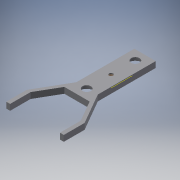
# Autodesk Inventor part: 28_Z_Stage
Saved by Autodesk Inventor 2016 (Build 200138000, 138)
## iProperties
Created: 2017-01-03
Part Number: 28_Z_Stage
Material: Generisch
Document SubType Name: Modeling
Designer: Bene
Density: 1 g/cm^3
Appearance: Vorgabe
Author: Bene
Autodesk Inventor part; units mm, degrees
ref_plane "YZ Plane" through (0, 0, 0) normal (1, 0, 0) x (0, 1, 0)
ref_plane "XZ Plane" through (0, 0, 0) normal (0, 1, 0) x (-1, 0, 0)
ref_plane "Arbeitsebene1" through (-1.3943, 18.6513, 4.1) normal (0, 0, 1) x (1, 0, 0)
sketch "Skizze1" plane through (-1.3943, 18.6513, 4.1) normal (0, 0, 1) x (1, 0, 0)
  circle A0 centre (1.3943, 6.3487) radius 8 projected
  circle A1 centre (1.3942, -43.6513) radius 8 projected
  circle A2 centre (1.3943, 6.3487) radius 8.3
  circle A3 centre (1.3942, -43.6513) radius 8.3
  circle A4 centre (1.3943, -18.6513) radius 1.5706 projected
  circle A5 centre (1.3943, -18.6513) radius 2.0706
  circle A6 centre (2.1966, -75.6683) radius 18 construction
  line L0 (14.0323, -55.1683) -> (-9.6391, -55.1683) construction
  line L1 (-9.6391, -55.1683) -> (-21.4748, -75.6683) construction
  line L2 (-21.4748, -75.6683) -> (-9.6391, -96.1683) construction
  line L3 (-9.6391, -96.1683) -> (14.0323, -96.1683) construction
  line L4 (14.0323, -96.1683) -> (25.8679, -75.6683) construction
  line L5 (25.8679, -75.6683) -> (14.0323, -55.1683) construction
  line L6 (12.3943, 16.3487) -> (-9.6057, 16.3487) construction
  line L7 (-9.6057, 16.3487) -> (-9.6057, -53.6513) construction
  line L8 (-9.6057, -53.6513) -> (12.3943, -53.6513) construction
  line L9 (12.3943, -53.6513) -> (12.3943, 16.3487) construction
  line L10 (12.3943, 16.3487) -> (-9.6057, -53.6513) construction
  line L11 (-9.6057, 16.3487) -> (12.3943, -53.6513) construction
  line L12 (12.3943, 16.3487) -> (-9.6057, 16.3487)
  line L13 (-9.6057, 16.3487) -> (-9.6057, -53.6513)
  line L14 (-9.6057, -53.6513) -> (12.3943, -53.6513)
  line L15 (12.3943, -53.6513) -> (12.3943, 16.3487)
  circle A7 centre (2.1966, -75.6683) radius 18 projected
  line L16 (14.0323, -55.1683) -> (-9.6391, -55.1683) construction
  line L17 (-9.6391, -55.1683) -> (-21.4748, -75.6683) construction
  line L18 (-21.4748, -75.6683) -> (-9.6391, -96.1683) construction
  line L19 (-9.6391, -96.1683) -> (14.0323, -96.1683) construction
  line L20 (14.0323, -96.1683) -> (25.8679, -75.6683) construction
  line L21 (25.8679, -75.6683) -> (14.0323, -55.1683) projected
  line L22 (14.321, -54.6683) -> (26.4453, -75.6683)
  line L23 (26.4453, -75.6683) -> (14.3209, -96.6683)
  line L24 (14.3209, -96.6683) -> (-9.9278, -96.6683)
  line L25 (-9.9278, -96.6683) -> (-22.0521, -75.6683)
  line L26 (-22.0521, -75.6683) -> (-9.9278, -54.6683)
  line L27 (-9.9278, -54.6683) -> (14.321, -54.6683)
  line L28 (12.3943, -53.6513) -> (14.3943, -53.6513)
  line L29 (14.3943, -53.6513) -> (26.8943, -75.3019)
  line L30 (26.8943, -75.3019) -> (26.8943, -96.6683)
  line L31 (26.8943, -96.6683) -> (30.8943, -96.6683)
  line L32 (30.8943, -96.6683) -> (30.8943, -75.3019)
  line L33 (30.8943, -75.3019) -> (12.3943, -43.259)
  line L34 (-9.6057, -53.6513) -> (-11.6057, -53.6513)
  line L35 (-11.6057, -53.6513) -> (-24.3173, -75.6683)
  line L36 (-24.3173, -75.6683) -> (-24.3173, -96.6683)
  line L37 (-24.3173, -96.6683) -> (-28.3173, -96.6683)
  line L38 (-28.3173, -96.6683) -> (-28.3173, -75.6683)
  line L39 (-28.3173, -75.6683) -> (-9.6057, -43.259)
  point P0 (1.3943, -18.6513)
  dimension "d0" = 0.3
  dimension "d1" = 0.3
  dimension "d2" = 0.5
  dimension "d3" = 22
  dimension "d4" = 70
  dimension "d7" = 0.5
  dimension "d8" = 2
  dimension "d9" = 25
  dimension "d10" = 120
  dimension "d11" = 4
  dimension "d12" = 2
  dimension "d13" = 120
  dimension "d14" = 4
  constraints: 56 end point, 8 perpendicular, 6 parallel, 5 point on line, 3 centre point, 2 horizontal, 2 midpoint, 5 other
  measures "d0" radial gap between concentric circles of A0 A2
  measures "d1" radial gap between concentric circles of A1 A3
  measures "d2" radial gap between concentric circles of A4 A5
  measures "d3" distance of L8.end L7.end
  measures "d4" distance of L7.end L6.end
  measures "d7" distance between parallel lines of L5 L22
  measures "d8" distance of L14.end L28.end
  measures "d9" distance of L28.end L29.end
  measures "d10" angle of L28 L29
  measures "d11" distance of L30.end L31.end
  measures "d12" distance of L7.end L34.end
  measures "d13" angle of L35 L34
  measures "d14" distance of L36.end L37.end
ref_plane "Arbeitsebene2" through (-16.3, -16.3, -1) normal (0, 0, 1) x (1, 0, 0)
extrude "Extrusion1" add sketch "Skizze1" against normal up to surface (5.1 mm away) contours L15 L14 L13 L12 | L33 L32 L31 L30 L29 L28 L15 | L13 L34 L35 L36 L37 L38 L39
sketch "Skizze2" plane through (-1.3943, 18.6513, 4.1) normal (0, 0, 1) x (1, 0, 0)
  circle A0 centre (1.3942, -43.6513) radius 8.3 projected
  circle A1 centre (1.3943, 6.3487) radius 8.3 projected
  circle A2 centre (1.3943, -18.6513) radius 2.0706 projected
  line L0 (-9.6057, -43.259) -> (-28.3173, -75.6683) projected
  line L1 (-28.3173, -75.6683) -> (-28.3173, -96.6683) projected
  line L2 (-28.3173, -96.6683) -> (-24.3173, -96.6683) projected
  line L3 (-24.3173, -96.6683) -> (-24.3173, -75.6683) projected
  line L4 (-24.3173, -75.6683) -> (-11.6057, -53.6513) projected
  line L5 (-11.6057, -53.6513) -> (14.3943, -53.6513) projected
  line L6 (14.3943, -53.6513) -> (26.8943, -75.3019) projected
  line L7 (26.8943, -75.3019) -> (26.8943, -96.6683) projected
  line L8 (26.8943, -96.6683) -> (30.8943, -96.6683) projected
  line L9 (30.8943, -96.6683) -> (30.8943, -75.3019) projected
  line L10 (30.8943, -75.3019) -> (12.3943, -43.259) projected
  line L11 (12.3943, -43.259) -> (12.3943, 16.3487) projected
  line L12 (12.3943, 16.3487) -> (-9.6057, 16.3487) projected
  line L13 (-9.6057, 16.3487) -> (-9.6057, -43.259) projected
  circle A3 centre (1.3943, 6.3487) radius 4 projected
  circle A4 centre (1.3942, -43.6513) radius 4 projected
  circle A5 centre (1.3943, 6.3487) radius 4.3
  circle A6 centre (1.3942, -43.6513) radius 4.3
  point P0 (1.3943, -18.6513)
  dimension "d15" = 0.3
  dimension "d16" = 0.3
  constraints: 2 centre point
  measures "d15" radial gap between concentric circles of A3 A5
  measures "d16" radial gap between concentric circles of A4 A6
extrude "Extrusion2" add sketch "Skizze2" along normal blind 1 contours A0 | A1 | L13 L12 L11 L10 L9 L8 L7 L6 L5 L4 L3 L2 L1 L0
